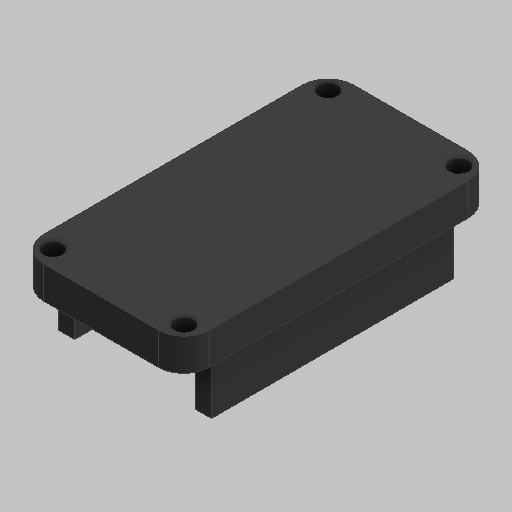
# Autodesk Inventor part: ESP_8266
Saved by Autodesk Inventor 2025 (Build 290162010, 162A)
## iProperties
Created: 2024-06-08
Part Number: ESP_8266
Material: Genérico
Document SubType Name: Sheet Metal
Designer: juesr
Density: 1 g/cm^3
Sheet Metal Rule: Por defecto_mm
Appearance: Valor por defecto
Author: juesr
Autodesk Inventor part; units mm, degrees
ref_plane "YZ Plane" through (0, 0, 0) normal (1, 0, 0) x (0, 1, 0)
ref_plane "XZ Plane" through (0, 0, 0) normal (0, 1, 0) x (-1, 0, 0)
ref_plane "XY Plane" through (0, 0, 0) normal (0, 0, 1) x (1, 0, 0)
sketch "Boceto1" plane through (0, 0, 0) normal (0, 1, 0) x (-1, 0, 0)
  line L0 (12.565, 24) -> (-13.135, 24)
  line L1 (-13.135, 24) -> (-13.135, -24)
  line L2 (-13.135, -24) -> (12.565, -24)
  line L3 (12.565, -24) -> (12.565, 24)
  point P0 (0, 0)
  point P1 (-0.285, -24)
  dimension "d0" = 48
  dimension "d1" = 25.7
  dimension "d2" = 12.565
  dimension "d3" = 24
  constraints: 8 end point, 2 parallel, 1 horizontal, 1 midpoint, 1 perpendicular
  measures "d0" distance between parallel lines of L2 L0
  measures "d1" distance between parallel lines of L1 L3
  measures "d2" distance from line of L3 point (0, 0)
  measures "d3" vertical distance of point (-0.285, -24) point (0, 0)
extrude "Extrusión1" add sketch "Boceto1" along normal blind 5
fillet "Empalme1" radius 4 3 edges at (13.135, 2.5, 24) (13.135, 2.5, -24) (-12.565, 2.5, 24)
fillet "Empalme2" radius 4 1 edges at (-12.565, 2.5, -24)
sketch "Boceto2" plane through (0, 5, 0) normal (0, 1, 0) x (1, 0, 0)
  circle A0 centre (-9.865, -21.3) radius 1.5
  line L0 (-8.565, -24) -> (9.135, -24) projected
  line L1 (-12.565, 20) -> (-12.565, -20) projected
  line L2 (-31.929, 0) -> (35.0281, 0)
  circle A1 centre (-9.865, 21.3) radius 1.5
  line L3 (0.285, 24.6166) -> (0.285, -27.3805)
  circle A2 centre (10.435, -21.3) radius 1.5
  circle A3 centre (10.435, 21.3) radius 1.5
  line L4 (13.135, -20) -> (13.135, 20) projected
  line L5 (9.135, 24) -> (-8.565, 24) projected
  point P0 (0, 0)
  dimension "d8" = 3
  dimension "d9" = 2.7
  dimension "d10" = 2.7
  dimension "d21" = 2.7
  dimension "d22" = 2.7
  constraints: 4 centre point, 4 end point, 3 symmetric about line, 1 horizontal, 1 vertical, 3 other
  measures "d8" diameter of A0
  measures "d9" distance from line of L0 A0.centre
  measures "d10" distance from line of L1 A0.centre
  measures "d21" distance from line of L4 A2.centre
  measures "d22" distance from line of L5 A3.centre
extrude "Extrusión2" cut sketch "Boceto2" against normal blind 10
sketch "Boceto3" plane through (0, 0, 0) normal (0, -1, 0) x (1, 0, 0)
  line L0 (-11.565, 18.75) -> (-9.065, 18.75)
  line L1 (-9.065, 18.75) -> (-9.065, -18.75)
  line L2 (-9.065, -18.75) -> (-11.565, -18.75)
  line L3 (-11.565, -18.75) -> (-11.565, 18.75)
  line L4 (0.285, 27.3547) -> (0.285, -28.7593)
  line L5 (-12.565, -20) -> (-12.565, 20) projected
  line L6 (-8.565, 24) -> (9.135, 24) projected
  line L7 (9.135, -24) -> (-8.565, -24) projected
  line L8 (12.135, 18.75) -> (9.635, 18.75)
  line L9 (9.635, 18.75) -> (9.635, -18.75)
  line L10 (9.635, -18.75) -> (12.135, -18.75)
  line L11 (12.135, -18.75) -> (12.135, 18.75)
  line L12 (13.135, 20) -> (13.135, -20) projected
  point P0 (0, 0)
  point P1 (-10.315, 18.75)
  point P2 (-10.315, -18.75)
  point P3 (10.885, 18.75)
  point P4 (10.885, -18.75)
  dimension "d13" = 37.5
  dimension "d14" = 2.5
  dimension "d15" = 1
  dimension "d16" = 5.25
  dimension "d17" = 5.25
  dimension "d18" = 1
  constraints: 18 end point, 6 symmetric about line, 2 midpoint, 2 parallel, 1 horizontal, 1 perpendicular, 1 vertical
  measures "d13" distance of point (-10.315, 18.75) point (-10.315, -18.75)
  measures "d14" distance between parallel lines of L1 L3
  measures "d15" distance between parallel lines of L5 L3
  measures "d16" distance from line of L6 point (-10.315, 18.75)
  measures "d17" distance from line of L7 point (-10.315, -18.75)
  measures "d18" distance between parallel lines of L12 L11
extrude "Extrusión3" add sketch "Boceto3" along normal blind 8
equation "\"Radio_pliegue\" = Grosor"
equation "\"Anchura_desahogo_plegado\" = Grosor"
equation "\"Profundidad_desahogo_plegado\" = 0.5 * Grosor"
equation "\"Tamaño_destalonado\" = 4 * Grosor"
equation "\"Remanente_mínimo\" = 2 * Grosor"
equation "\"Radiodetransición\" = Radio_pliegue"
equation "\"Tamaño_de_radio_de_Jacobi\" = Radio_pliegue"
equation "\"TamañoSeparación\" = Grosor"
equation "\"Grosor\" = 0.5"
